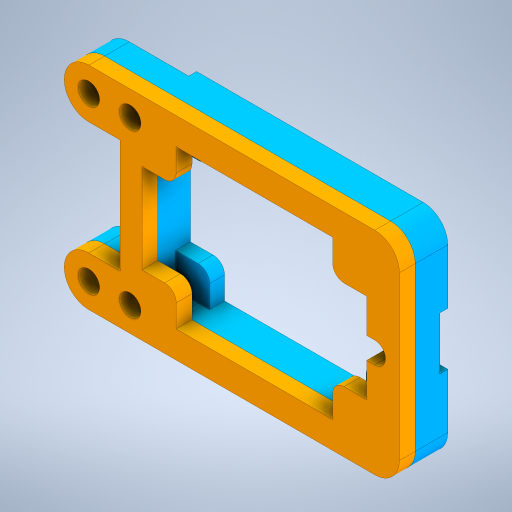
# Autodesk Inventor part: IMU Holder
Saved by Autodesk Inventor 2023 (Build 270158000, 158)
## iProperties
Created: 2022-07-03
Part Number: IMU Holder
Material: Generic
Document SubType Name: Modeling
Designer: Jochen Alt
Density: 1 g/cm^3
Appearance: Default
Author: Jochen Alt
Autodesk Inventor part; units mm, degrees
ref_plane "YZ Plane" through (0, 0, 0) normal (1, 0, 0) x (0, 1, 0)
ref_plane "XZ Plane" through (0, 0, 0) normal (0, 1, 0) x (-1, 0, 0)
ref_plane "XY Plane" through (0, 0, 0) normal (0, 0, 1) x (1, 0, 0)
sketch "Sketch1" plane through (0, 0, 0) normal (0, 0, 1) x (1, 0, 0)
  line L0 (-38.4722, 0) -> (38.4722, 0) construction
  line L1 (0, -24.3263) -> (0, 25.1372) construction
  line L2 (-27.4801, 0) -> (27.4801, 0) construction
  line L3 (0, -17.2601) -> (0, 18.071) construction
  line L4 (-16.256, 12.0396) -> (-12.4968, 12.0396)
  line L5 (19.05, 9.2456) -> (19.05, -9.2456)
  line L6 (16.256, -12.0396) -> (-12.4968, -12.0396)
  line L7 (-19.05, -9.2456) -> (-19.05, 9.2456) construction
  line L8 (-16.256, 9.2456) -> (-16.256, -9.2456) construction
  circle A0 centre (-16.256, 9.2456) radius 1.2192
  circle A1 centre (-16.256, -9.2456) radius 1.2192
  arc A2 (16.256, -1.2192) -> (16.256, 1.2192) centre (16.256, 0) ccw
  arc A3 (-16.256, 12.0396) -> (-19.05, 9.2456) centre (-16.256, 9.2456) ccw construction
  arc A4 (-19.05, -9.2456) -> (-16.256, -12.0396) centre (-16.256, -9.2456) ccw
  arc A5 (16.256, -12.0396) -> (19.05, -9.2456) centre (16.256, -9.2456) ccw
  arc A6 (19.05, 9.2456) -> (16.256, 12.0396) centre (16.256, 9.2456) ccw
  line L9 (-16.256, 9.2456) -> (-12.4968, 9.2456) construction
  line L10 (-12.4968, 6.4516) -> (-12.7, 6.4516)
  arc A7 (-16.256, 12.0396) -> (-16.256, 6.4516) centre (-16.256, 9.2456) ccw
  arc A8 (-12.4968, 6.4516) -> (-12.4968, 12.0396) centre (-12.4968, 9.2456) ccw
  line L11 (-16.256, -9.2456) -> (-12.4968, -9.2456) construction
  line L12 (-12.4968, -6.4516) -> (-16.256, -6.4516)
  arc A9 (-16.256, -6.4516) -> (-19.05, -9.2456) centre (-16.256, -9.2456) ccw
  arc A10 (-12.4968, -12.0396) -> (-12.4968, -6.4516) centre (-12.4968, -9.2456) ccw
  circle A11 centre (-11.556, 9.2456) radius 1.2192
  circle A12 centre (-11.556, -9.2456) radius 1.2192
  line L13 (-11.556, 9.2456) -> (-11.556, -9.2456) construction
  line L14 (-12.7, 6.4516) -> (-12.7, -6.4516)
  circle A13 centre (16.256, 0) radius 2.794
  arc A14 (-12.4968, 12.0396) -> (-12.4968, 6.4516) centre (-12.4968, 9.2456) ccw
  arc A15 (-12.4968, -6.4516) -> (-15.217, -8.6077) centre (-12.4968, -9.2456) ccw
  line L15 (-12.4968, 12.0396) -> (16.256, 12.0396)
  line L16 (-12.4968, -12.0396) -> (-16.256, -12.0396)
  line L17 (-12.7, 6.4516) -> (-16.256, 6.4516)
  arc A16 (-15.217, -8.6077) -> (-12.4968, -12.0396) centre (-12.4968, -9.2456) ccw
  line L18 (-7.64, 8.965) -> (12.79, 8.965)
  line L19 (15.35, 6.405) -> (15.35, -6.405)
  line L20 (12.79, -8.965) -> (-7.64, -8.965)
  line L21 (-10.2, -6.405) -> (-10.2, 6.405)
  arc A17 (-7.64, 8.965) -> (-10.2, 6.405) centre (-7.64, 6.405) ccw
  arc A18 (15.35, 6.405) -> (12.79, 8.965) centre (12.79, 6.405) ccw
  arc A19 (12.79, -8.965) -> (15.35, -6.405) centre (12.79, -6.405) ccw
  arc A20 (-10.2, -6.405) -> (-7.64, -8.965) centre (-7.64, -6.405) ccw
  circle A21 centre (-12.4968, -9.2456) radius 2.994
  circle A22 centre (16.256, 0) radius 2.994
  circle A23 centre (-12.4968, 9.2456) radius 2.994
  circle A24 centre (-7.64, 6.405) radius 1.215
  circle A25 centre (-7.64, -6.405) radius 1.215
  circle A26 centre (12.79, 6.405) radius 1.215
  circle A27 centre (12.79, -6.405) radius 1.215
  arc A28 (-6.325, -6.405) -> (-7.64, -5.09) centre (-7.64, -6.405) ccw
  arc A29 (12.79, -5.09) -> (11.475, -6.405) centre (12.79, -6.405) ccw
  arc A30 (11.475, 6.405) -> (12.79, 5.09) centre (12.79, 6.405) ccw
  arc A31 (-7.64, 5.09) -> (-6.325, 6.405) centre (-7.64, 6.405) ccw
  line L22 (-7.64, -5.09) -> (-10.2, -5.09)
  line L23 (-7.64, 5.09) -> (-10.2, 5.09)
  line L24 (-6.325, -6.405) -> (-6.325, -8.965)
  line L25 (11.475, -6.405) -> (11.475, -8.965)
  line L26 (12.79, -5.09) -> (15.35, -5.09)
  line L27 (12.79, 5.09) -> (15.35, 5.09)
  line L28 (11.475, 6.405) -> (11.475, 8.965)
  line L29 (-6.325, 6.405) -> (-6.325, 8.965)
  line L30 (16.256, -1.2192) -> (15.35, -1.2192)
  line L31 (16.256, 1.2192) -> (15.35, 1.2192)
  line L32 (16.256, 2.994) -> (19.05, 2.994)
  line L33 (16.256, -2.994) -> (19.05, -2.994)
  line L34 (-9.5028, -9.2456) -> (-9.5028, -12.0396)
  line L35 (-9.5028, 9.2456) -> (-9.5028, 12.0396)
  point P0 (-19.05, -9.2456)
  point P1 (-19.05, 9.2456)
  point P2 (0, 0)
  point P3 (19.05, -12.0396)
  point P4 (19.05, 12.0396)
  point P5 (-19.05, -12.0396)
  point P6 (-14.3764, 9.2456)
  point P7 (-14.3764, -9.2456)
  point P8 (-19.05, -9.2456)
  point P9 (-19.05, 9.2456)
  point P10 (0, 0)
  point P11 (-10.2, 8.965)
  point P12 (-10.2, -8.965)
  point P13 (19.05, 0)
  point P14 (15.0532, -0.1993)
  point P15 (15.0532, 0.1993)
  point P16 (-11.4209, 12.0396)
  point P17 (-9.6552, 8.3026)
  point P18 (15.35, 2.643)
  point P19 (19.05, -1.0759)
  point P20 (19.05, 1.0759)
  point P21 (15.35, -2.8536)
  point P22 (-9.6552, -8.3026)
  point P23 (-11.4209, -12.0396)
  point P24 (-10.3976, 7.1108)
  point P25 (-12.7, 6.2585)
  point P26 (-12.7, -6.2585)
  point P27 (-10.3976, -7.1108)
  point P28 (-13.5727, -6.4516)
  point P29 (15.35, 2.8536)
  point P30 (-19.05, -9.2456)
  point P31 (-15.217, -9.8835)
  point P32 (-7.8539, 8.956)
  point P33 (-15.371, -10.0842)
  dimension "d9" = 38.1
  dimension "d10" = 24.0792
  dimension "d11" = 18.4912
  dimension "d12" = 2.4384
  dimension "d13" = 32.512
  dimension "d14" = 3.7592
  dimension "d15" = 4.7
  dimension "d16" = 6.35
  dimension "d20" = 17.93
  dimension "d21" = 25.55
  dimension "d22" = 2.56
  dimension "d25" = 0.2
  dimension "d26" = 2.43
  dimension "d30" = 0.1
  dimension "d33" = 10.2
  constraints: 72 end point, 47 tangent, 43 point on circle, 37 point on line, 29 centre point, 18 perpendicular, 15 coincident, 14 equal radius, 10 parallel, 3 horizontal, 3 midpoint, 2 concentric, 2 vertical, 16 other
  measures "d9" distance of point (19.05, -12.04) point (-19.05, -12.04)
  measures "d10" distance of point (19.05, 12.04) point (19.05, -12.04)
  measures "d11" distance of L8.start L8.end
  measures "d12" diameter of A0
  measures "d13" distance from line of A2.centre L8
  measures "d14" distance of L9.end L8.start
  measures "d15" distance of L13.start L8.start
  measures "d16" distance between parallel lines of L14 L7
  measures "d20" distance of point (-10.2, -8.965) point (-10.2, 8.965)
  measures "d21" distance between parallel lines of L19 L21
  measures "d22" radius of A17
  measures "d26" diameter of A24
  measures "d30" radial gap between concentric circles of A24 A31
  measures "d33" distance between parallel lines of L3 L21
extrude "Extrusion1" add sketch "Sketch1" along normal blind 2.8 contours L4 A23 A0 L17 A7 | L4 A14 A0 A23 | L15 A23 L14 L10 A8 | A8 A14 A0 | L15 L35 A23 | A23 A0 A14 L10 L17 | L15 A6 L5 L32 A22 L19 A18 L18 A17 L21 A20 L20 A19 L33 A5 L6 L34 A21 L14 A23 L35 | A21 L6 A10 L12 L14 | L12 A15 A1 A21 | L34 L6 A21 | A21 A1 L16 A4 A9 L12 | L5 A22 L32 | A10 A16 A1 A15 | L5 A13 L19 A22 | L16 A21 A1 A16 | A13 L19 L30 A2 L31 | L5 A22 L19 A13 | L5 L33 A22
extrude "Extrusion2" add sketch "Sketch1" along normal blind 0.8 and the other way blind 0.9 contours L15 A6 L5 L32 A22 L19 A18 L18 A17 L21 A20 L20 A19 L33 A5 L6 L34 A21 L14 A23 L35 | L27 A30 L28 L18 A18 L19 | L19 A19 L20 L25 A29 L26 | L29 A31 L23 L21 A17 L18 | L20 A20 L21 L22 A28 L24 | A24 | A25 | A26 | A27
extrude "Extrusion3" add sketch "Sketch1" along normal blind 1.8 from surface at 2.8 separate body contours L4 A23 A0 L17 A7 | L4 A14 A0 A23 | L15 A23 L14 L10 A8 | A8 A14 A0 | L15 L35 A23 | A23 A0 A14 L10 L17 | L15 A6 L5 L32 A22 L19 A18 L18 A17 L21 A20 L20 A19 L33 A5 L6 L34 A21 L14 A23 L35 | A21 L6 A10 L12 L14 | L12 A15 A1 A21 | L34 L6 A21 | A21 A1 L16 A4 A9 L12 | L5 A22 L32 | A10 A16 A1 A15 | L5 A13 L19 A22 | L16 A21 A1 A16 | A13 L19 L30 A2 L31 | L5 A22 L19 A13 | L5 L33 A22 | L27 A30 L28 L18 A18 L19 | L19 A19 L20 L25 A29 L26 | L29 A31 L23 L21 A17 L18 | L20 A20 L21 L22 A28 L24 | A24 | A25 | A26 | A27
